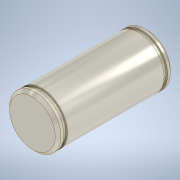
# Autodesk Inventor part: pin_stempel_stang
Saved by Autodesk Inventor 2022 (Build 260153000, 153)
## iProperties
Created: 2022-04-10
Part Number: pin_stempel_stang
Material: Titanium
Document SubType Name: Modeling
Designer: Patrick
Density: 4.51 g/cm^3
Appearance: Titanium
Mass: 46.4363 g
Surface Area: 28.5911 cm^2
Volume: 10.2963 cm^3
Author: Patrick
Autodesk Inventor part; units mm, degrees
ref_plane "YZ Plane" through (0, 0, 0) normal (1, 0, 0) x (0, 1, 0)
ref_plane "XZ Plane" through (0, 0, 0) normal (0, 1, 0) x (-1, 0, 0)
ref_plane "XY Plane" through (0, 0, 0) normal (0, 0, 1) x (1, 0, 0)
sketch "Sketch1" plane through (0, 0, 0) normal (0, 1, 0) x (-1, 0, 0)
  line L0 (0, 0) -> (9, 0)
  line L1 (9, 0) -> (9, -17)
  line L2 (9, -17) -> (8.5, -17)
  line L3 (8.5, -17) -> (8.5, -18.2)
  line L4 (8.5, -18.2) -> (9, -18.2)
  line L5 (9, -18.2) -> (9, -19.2)
  line L6 (9, -19.2) -> (8, -20.2)
  line L7 (8, -20.2) -> (0, -20.2)
  line L8 (0, -20.2) -> (0, 0)
  line L9 (9, 0) -> (9, 17)
  line L10 (8.5, 17) -> (8.5, 18.2)
  line L11 (8.5, 18.2) -> (9, 18.2)
  line L12 (9, 18.2) -> (9, 19.2)
  line L13 (9, 19.2) -> (8, 20.2)
  line L14 (8, 20.2) -> (0, 20.2)
  line L15 (0, 20.2) -> (0, 0)
  line L16 (9, 17) -> (8.5, 17)
  dimension "d0" = 2
  dimension "d2" = 1.2
  dimension "d3" = 1
  dimension "d4" = 135
  dimension "d5" = 9
  dimension "d7" = 17
  dimension "d11" = 0.5
  constraints: 34 end point, 7 symmetric about line, 5 perpendicular, 4 point on line, 2 horizontal, 1 parallel
  measures "d0" distance between parallel lines of L7 L4
  measures "d2" distance of L2.end L3.end
  measures "d3" horizontal distance of L6.end L5.end
  measures "d4" angle of L5 L6
  measures "d5" distance between parallel lines of L8 L1
  measures "d7" distance of L0.end L1.end
  measures "d11" distance of L1.end L2.end
revolve "Revolution1" add sketch "Sketch1" angle 360 about axis through (0, 0, 20.2) along (0, 0, -1)
body "Solid1"
